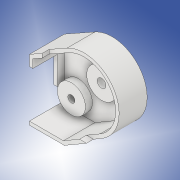
# Autodesk Inventor part: BA005
Saved by Autodesk Inventor 2017 (Build 210142000, 142)
## iProperties
Created: 2017-06-15
Part Number: BA005
Material: ABS Plastic
Document SubType Name: Modeling
Designer: zallen
Density: 1.06 g/cm^3
Appearance: CR White
Author: zallen
Autodesk Inventor part; units mm, degrees
ref_plane "YZ Plane" through (0, 0, 0) normal (1, 0, 0) x (0, 1, 0)
ref_plane "XZ Plane" through (0, 0, 0) normal (0, 1, 0) x (-1, 0, 0)
ref_plane "XY Plane" through (0, 0, 0) normal (0, 0, 1) x (1, 0, 0)
sketch "Sketch1" plane through (0, 0, 0) normal (0, 0, 1) x (1, 0, 0)
  line L0 (0, 0) -> (0, 87.5)
  line L1 (0, 87.5) -> (43.6046, 111.967)
  line L2 (0, 0) -> (50, 0)
  line L3 (50, 0) -> (93.217, 25.1454)
  circle A0 centre (68.0717, 68.3624) radius 50 construction
  arc A1 (93.217, 25.1454) -> (43.6046, 111.967) centre (68.0717, 68.3624) ccw
  dimension "d0" = 87.5
  dimension "d1" = 50
  dimension "d2" = 50
  dimension "d3" = 50
  dimension "d4" = 100
  constraints: 8 end point, 4 point on circle, 3 tangent, 2 centre point, 1 concentric, 1 horizontal, 1 vertical
  measures "d0" distance of L0.start L0.end
  measures "d1" distance of L0.end L1.end
  measures "d2" distance of L0.start L2.end
  measures "d3" distance of L2.end L3.end
  measures "d4" diameter of A0
extrude "Extrusion1" add sketch "Sketch1" along normal blind 50
sketch "Sketch2" plane through (0, 0, 50) normal (0, 0, 1) x (1, 0, 0)
  line L0 (0, 0) -> (50, 0) projected
  line L1 (50, 0) -> (93.217, 25.1454) projected
  arc A0 (93.217, 25.1454) -> (43.6046, 111.967) centre (68.0717, 68.3624) ccw projected
  line L2 (43.6046, 111.967) -> (0, 87.5) projected
  line L3 (0, 81.7667) -> (46.0513, 107.6066)
  arc A1 (90.7025, 29.4671) -> (46.0513, 107.6066) centre (68.0717, 68.3624) ccw
  line L4 (90.7025, 29.4671) -> (48.6512, 5)
  line L5 (48.6512, 5) -> (0, 5)
  line L6 (0, 87.5) -> (0, 0) projected
  line L7 (0, 5) -> (0, 81.7667)
  dimension "d7" = 5
  constraints: 8 end point, 2 point on circle, 1 centre point, 1 collinear, 1 point on line, 3 other
  measures "d7" distance between parallel lines of L1 L4
extrude "Extrusion2" cut sketch "Sketch2" against normal blind 45 contours L6 L3 A1 L4 L5
sketch "Sketch3" plane through (0, 0, 0) normal (-1, 0, 0) x (0, 0, 1)
  line L0 (0, 87.5) -> (50, 87.5) projected
  line L1 (50, 113.3624) -> (50, 29.4671) projected
  line L2 (0, 87.5) -> (50, 87.5)
  line L3 (50, 87.5) -> (50, 72.5)
  line L4 (50, 72.5) -> (0, 72.5)
  line L5 (0, 72.5) -> (0, 87.5)
  point P0 (0, 0)
  point P1 (50, 107.6066)
  dimension "d10" = 15
  constraints: 8 end point, 2 parallel, 1 horizontal, 1 perpendicular, 1 point on line
  measures "d10" distance of L2.end L3.end
extrude "Extrusion3" add sketch "Sketch3" against normal blind 5
sketch "Sketch4" plane through (0, 0, 0) normal (-1, 0, 0) x (0, 0, 1)
  line L0 (0, 87.5) -> (0, 111.967) projected
  line L1 (0, 87.5) -> (15, 87.5)
  line L2 (15, 87.5) -> (15, 32.5)
  line L3 (15, 32.5) -> (0, 32.5)
  line L4 (0, 32.5) -> (0, 87.5)
  line L5 (0, 0) -> (50, 0) projected
  dimension "d13" = 15
  dimension "d14" = 32.5
  constraints: 8 end point, 2 parallel, 1 horizontal, 1 perpendicular
  measures "d13" distance of L2.end L3.end
  measures "d14" distance between parallel lines of L5 L3
extrude "Extrusion4" add sketch "Sketch4" against normal blind 5
sketch "Sketch6" plane through (0, 0, 5) normal (0, 0, 1) x (1, 0, 0)
  circle A0 centre (25, 27.5) radius 20
  line L0 (48.6512, 5) -> (0, 5) projected
  line L1 (0, 5) -> (0, 32.5) projected
  circle A1 centre (25, 27.5) radius 5
  point P0 (0, 0)
  dimension "d22" = 40
  dimension "d37" = 22.5
  dimension "d38" = 25
  dimension "d39" = 10
  constraints: 2 centre point, 1 coincident
  measures "d22" diameter of A0
  measures "d37" distance from line of A0.centre L0
  measures "d38" distance from line of L1 A0.centre
  measures "d39" diameter of A1
sketch "Sketch7" plane through (0, 0, 5) normal (0, 0, 1) x (1, 0, 0)
  arc A0 (93.217, 25.1454) -> (43.6046, 111.967) centre (68.0717, 68.3624) ccw projected
  circle A1 centre (68.0717, 68.3624) radius 6.25
  circle A2 centre (68.0717, 68.3624) radius 21.25
  point P0 (0, 0)
  dimension "d25" = 12.5
  dimension "d28" = 15
  constraints: 2 centre point, 1 coincident
  measures "d25" diameter of A1
  measures "d28" radial gap between concentric circles of A1 A2
extrude "Extrusion8" add sketch "Sketch7" along normal blind 10
sketch "Sketch8" plane through (68.0717, 68.3624, 5) normal (0, 0, 1) x (1, 0, 0)
  circle A0 centre (0, 0) radius 6.25 projected
  circle A1 centre (0, 0) radius 6.25
  point P0 (-68.0717, -68.3624)
  constraints: 1 centre point, 1 coincident
extrude "Extrusion9" cut sketch "Sketch8" against normal through all
sketch "Sketch9" plane through (0, 0, 0) normal (0, 0, -1) x (-1, 0, 0)
  circle A0 centre (-68.0717, 68.3624) radius 21.25 projected
  circle A1 centre (-68.0717, 68.3624) radius 21.25
  point P0 (0, 0)
  constraints: 1 centre point, 1 concentric
extrude "Extrusion10" add sketch "Sketch9" along normal blind 5
sketch "Sketch10" plane through (0, 0, 50) normal (0, 0, 1) x (1, 0, 0)
  arc A0 (93.217, 25.1454) -> (43.6046, 111.967) centre (68.0717, 68.3624) ccw projected
  circle A1 centre (68.0717, 68.3624) radius 50
  line L0 (18.0717, 68.3624) -> (18.0717, 97.6402)
  line L1 (0, 87.5) -> (43.6046, 111.967) projected
  line L2 (43.6046, 111.967) -> (18.0717, 97.6402)
  line L3 (68.0717, 18.3624) -> (81.5592, 18.3624)
  line L4 (50, 0) -> (93.217, 25.1454) projected
  line L5 (81.5592, 18.3624) -> (93.217, 25.1454)
  point P0 (0, 0)
  constraints: 8 end point, 4 tangent, 2 collinear, 2 point on circle, 2 point on line, 1 centre point, 1 coincident, 1 concentric, 1 vertical, 1 vertical alignment
extrude "Extrusion11" cut sketch "Sketch10" against normal blind 10
extrude "Extrusion12" add sketch "Sketch6" along normal blind 10
body "Solid1"
